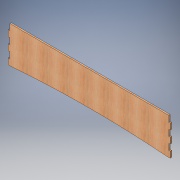
# Autodesk Inventor part: back
Saved by Autodesk Inventor 2016 (Build 200138000, 138)
## iProperties
Created: 2017-02-03
Part Number: back
Material: Wood (Birch)
Document SubType Name: Modeling
Designer: jwillauer
Density: 0.55 g/cm^3
Appearance: Birch - Natural Polished
Author: jwillauer
Autodesk Inventor part; units mm, degrees
ref_plane "YZ Plane" through (0, 0, 0) normal (1, 0, 0) x (0, 1, 0)
ref_plane "XZ Plane" through (0, 0, 0) normal (0, 1, 0) x (-1, 0, 0)
ref_plane "XY Plane" through (0, 0, 0) normal (0, 0, 1) x (1, 0, 0)
sketch "Sketch1" plane through (0, 0, 0) normal (0, 0, 1) x (1, 0, 0)
  line L0 (-998.1754, 340.1521) -> (1033.8246, 340.1521)
  line L1 (1033.8246, 340.1521) -> (1033.8246, -117.0479)
  line L2 (-998.1754, -117.0479) -> (-998.1754, 340.1521)
  arc A0 (995.7246, -117.0479) -> (-960.0754, -117.0479) centre (17.8246, -12647.7146) ccw
  line L3 (1033.8246, -117.0479) -> (995.7246, -117.0479)
  line L4 (-960.0754, -117.0479) -> (-998.1754, -117.0479)
  point P0 (0, 0)
  dimension "d0" = 2032
  dimension "d1" = 457.2
  constraints: 10 end point, 3 parallel, 2 point on circle, 1 centre point, 1 horizontal, 1 perpendicular
  measures "d0" distance of L0.start L0.end
  measures "d1" distance of L0.end L1.end
extrude "Extrusion1" add sketch "Sketch1" along normal blind 19.05
sketch "Sketch2" plane through (0, 0, 19.05) normal (0, 0, 1) x (1, 0, 0)
  line L0 (1033.8246, 340.1521) -> (-998.1754, 340.1521) projected
  line L1 (-998.1754, -117.0479) -> (-960.0754, -117.0479) projected
  line L2 (-998.1754, 340.1521) -> (-979.1254, 340.1521)
  line L3 (-979.1254, 340.1521) -> (-979.1254, -117.0479)
  line L4 (-979.1254, -117.0479) -> (-998.1754, -117.0479)
  line L5 (-998.1754, -117.0479) -> (-998.1754, 340.1521)
  line L6 (1033.8246, -117.0479) -> (1033.8246, 340.1521) projected
  line L7 (1033.8246, 340.1521) -> (1014.7746, 340.1521)
  line L8 (1014.7746, 340.1521) -> (1014.7746, -117.0479)
  line L9 (1014.7746, -117.0479) -> (1033.8246, -117.0479)
  line L10 (1033.8246, -117.0479) -> (1033.8246, 340.1521)
  line L11 (-998.1754, 340.1521) -> (-998.1754, -117.0479) projected
  line L12 (-998.1754, 263.9521) -> (-979.1254, 263.9521)
  line L13 (1014.7746, 263.9521) -> (1033.8246, 263.9521)
  line L14 (-998.1754, 187.7521) -> (-979.1254, 187.7521)
  line L15 (1014.7746, 187.7521) -> (1033.8246, 187.7521)
  line L16 (-998.1754, 111.5521) -> (-979.1254, 111.5521)
  line L17 (1014.7746, 111.5521) -> (1033.8246, 111.5521)
  line L18 (-998.1754, 35.3521) -> (-979.1254, 35.3521)
  line L19 (1014.7746, 35.3521) -> (1033.8246, 35.3521)
  line L20 (1033.8246, -40.8479) -> (1014.7746, -40.8479)
  line L21 (-979.1254, -40.8479) -> (-998.1754, -40.8479)
  point P0 (0, 0)
  dimension "d7" = 19.05
  dimension "d8" = 19.05
  constraints: 36 end point, 17 point on line, 12 perpendicular, 5 midpoint, 4 parallel, 2 horizontal
  measures "d7" distance between parallel lines of L3 L5
  measures "d8" distance between parallel lines of L6 L8
extrude "Extrusion2" cut sketch "Sketch2" against normal blind 19.05 contours L6 L13 L8 L0 | L6 L17 L8 L15 | L6 L20 L8 L19 | L3 L12 L5 L0 | L3 L16 L5 L14 | L3 L21 L5 L18
body "Solid1"
